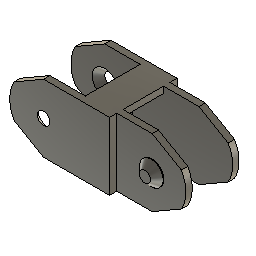
Cable Chain (Autodesk Fusion 360 design; units mm, degrees)
Autodesk Fusion 360 part; units mm, degrees
note: some values were not read from the file. Set by a fixed rule: which sketch regions a step uses.
sketch "Sketch1" plane through (0, 0, 0) normal (0, 1, 0) x (1, 0, 0) in component "Chain Link"
  line L0 (19.05, -10.3) -> (-19.05, -10.3)
  line L1 (-19.05, -10.3) -> (-19.05, 10.3)
  line L2 (-19.05, 10.3) -> (19.05, 10.3)
  line L3 (19.05, 10.3) -> (19.05, -10.3)
  line L4 (19.05, -10.3) -> (-19.05, 10.3) construction
  line L5 (-19.05, -10.3) -> (19.05, 10.3) construction
  line L6 (19.05, -12.7) -> (-19.05, -12.7)
  line L7 (-19.05, -12.7) -> (-19.05, 12.7)
  line L8 (-19.05, 12.7) -> (19.05, 12.7)
  line L9 (19.05, 12.7) -> (19.05, -12.7)
  line L10 (19.05, -12.7) -> (-19.05, 12.7) construction
  line L11 (-19.05, -12.7) -> (19.05, 12.7) construction
  arc A0 (-19.05, 12.7) -> (-19.05, -12.7) centre (-19.05, 0) ccw
  line L12 (-19.05, 0) -> (19.05, 0) construction
  arc A1 (19.05, 13.3) -> (19.05, -13.3) centre (19.05, 0) ccw construction
  circle A2 centre (-19.05, 0) radius 4.7625
  circle A3 centre (19.05, 0) radius 4.4625
  line L13 (19.05, -13.3) -> (19.05, 13.3) construction
  line L14 (0, 0) -> (0, -12.7) construction
  arc A4 (19.05, -12.7) -> (19.05, 12.7) centre (19.05, 0) ccw
  line L15 (-19.05, 12.7) -> (-30.0485, 6.35)
  line L16 (-19.05, -12.7) -> (-30.0485, -6.35)
  line L17 (19.05, -12.7) -> (30.0485, -6.35)
  line L18 (19.05, 12.7) -> (30.0485, 6.35)
  line L19 (5.75, -12.7) -> (5.75, 12.7)
  line L20 (-5.75, -12.7) -> (-5.75, 12.7)
  dimension "d7" = 38.1
  dimension "d9" = 2.4
  dimension "d11" = 0.6
  dimension "d12" = 9.525
  dimension "d13" = 8.925
  dimension "d63" = 25.4
  dimension "d66" = 60
  constraint horizontal L0
  constraint perpendicular L0 L1
  constraint parallel L0 L2
  constraint parallel L1 L3
  constraint coincident L4 L14.start
  constraint coincident L5 L14.start
  constraint coincident L14.start origin
  constraint horizontal L6
  constraint perpendicular L6 L7
  constraint parallel L6 L8
  constraint parallel L7 L9
  constraint coincident L10 L14.start
  constraint coincident L11 L14.start
  constraint equal L0 L6
  constraint tangent L6 A0
  constraint coincident A0.centre L12.start
  constraint midpoint L9 L12.end
  constraint symmetric L12 A1.start A1.end
  constraint coincident L12.end A1.centre
  constraint concentric A0 A2
  constraint concentric A1 A3
  constraint coincident L0.start L9
  constraint coincident L3 A1.end
  constraint vertical L13
  constraint coincident A1.start L13
  constraint coincident A0 L15.end
  constraint symmetric L7.end L12 L6.end
  constraint symmetric L12 L15.end L16.end
  constraint symmetric L7.end L14 L8.end
  constraint symmetric L14 L15.end L18.end
  constraint symmetric L14 L6.end L6.start
  constraint symmetric L14 L16.end L17.end
  constraint vertical L14
  constraint coincident L6 L14.end
  constraint coincident L8.end L9.start
  constraint coincident A1.end L13.start
  constraint coincident A1.start L13.end
  constraint tangent L6 A4
  constraint coincident L6 L19.start
  constraint coincident L8 L19.end
  constraint perpendicular L8 L19
  constraint tangent A1 L19
  constraint symmetric L14 L19.start L20.start
  constraint symmetric L14 L19.end L20.end
  measures "d7" distance of L1.end L2.end
  measures "d9" distance of L0 L6
  measures "d11" distance of L6 A1.end
  measures "d12" diameter of A2
  measures "d13" diameter of A3
  measures "d63" distance of L6 L8
  measures "d66" angle of L7 L15
extrude "Extrude1" add sketch "Sketch1" along normal blind 2.4 contours L0 L6 L19 L20 | L0 L2 L19 L20 | L3 L9 A3 | L3 L9 A3 | L0 L6 L7 L20 | L0 L1 L2 L7 A2 L20 | L2 L8 L19 L20 | L1 L7 A0 A2 L15 L16 | L2 L7 L8 L20 makes body 1 at (-0.9292, 2.4, 0) makes body 2 at (23.4903, 0.8, 0.4443) in component "Chain Link"
draft "Draft1" angle 45 neutral plane through (0, 2.4, 0) pull (0, 1, 0) 1 faces at (-14.2934, 1.6, 0.2374) on bodies 1 in component "Chain Link"
draft "Draft2" angle -45 neutral plane through (0, 2.4, 0) pull (0, 1, 0) 1 faces at (23.4903, 0.8, 0.4443) on bodies 2 in component "Chain Link"
extrude "Extrude4" add sketch "Sketch1" along normal blind 0.3 from surface at 2.4 contours L0 L6 L19 L20 | L0 L2 L19 L20 | L3 L9 A3 | L3 L9 A3 | L2 L8 L19 L20 bodies 1 2 in component "Chain Link"
extrude "Extrude2" add sketch "Sketch1" along normal blind 2.4 from surface at 2.7 contours L0 L6 L9 L19 | L0 L2 L3 L9 A3 L19 | L3 L9 A3 A4 L17 L18 | L0 L6 L19 L20 | L0 L2 L19 L20 | L3 L9 A3 | L3 L9 A3 | L2 L8 L9 L19 | L2 L8 L19 L20 bodies 1 2 in component "Chain Link"
extrude "Extrude3" add sketch "Sketch1" along normal blind 12.7 contours L0 L6 L19 L20 | L2 L8 L19 L20 bodies 1 in component "Chain Link"
mirror "Mirror1" about plane through (0, 12.7, 0) normal (0, 1, 0) of bodies 1 merged in component "Chain Link"
component "Chain Link" placed x (1, 0, 0) y (0, 1, 0) z (0, 0, 1) at (0, 0, 0)
equation "WIDTH = 1 in" comment "Internal Width"
equation "HEIGHT = 1 in" comment "Internal Height"
equation "WALL = 2.4 mm" comment "Wall thickness (some multiple of nozzle/layer thickness)"
equation "LENGTH = 1.5 in" comment "Joint-Joint Distance"
equation "d7 = LENGTH"
equation "d9 = WALL"
equation "AXLE_TOLERANCE = NOZZLE" comment "Fit tolerance of link joint axles"
equation "d11 = AXLE_TOLERANCE"
equation "d12 = AXLE_DIAMETER"
equation "d13 = AXLE_DIAMETER - AXLE_TOLERANCE"
equation "d14 = WALL"
equation "d19 = WALL"
equation "d21 = WIDTH / 2"
equation "d27 = AXLE_DRAFT"
equation "d29 = -AXLE_DRAFT"
equation "NOZZLE = 0.6 mm" comment "Nozzle Diameter"
equation "LINK_TOLERANCE = 0.3 mm" comment "Wiggle tolerance for links"
equation "d43 = LINK_TOLERANCE"
equation "d63 = HEIGHT"
equation "AXLE_DIAMETER = min(HEIGHT / 1.5; 0.375 in)"
equation "AXLE_DRAFT = 45 deg"
equation "d66 = PRINTER_OVERHANG"
equation "PRINTER_OVERHANG = 60 deg"
